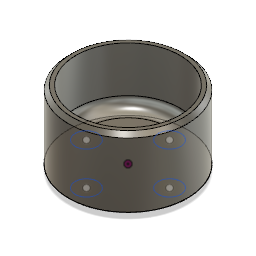
candle_holder (Autodesk Fusion 360 design; units mm, degrees)
Autodesk Fusion 360 part; units mm, degrees
note: some values were not read from the file. Set by a fixed rule: which face or edge a step refers to.
sketch "Sketch1" plane through (0, 0, 0) normal (0, 1, 0) x (1, 0, 0)
  circle A0 centre (0, 0) radius 31.75
  dimension "d6" = 63.5
  measures "d6" diameter of A0
extrude "Extrude1" add sketch "Sketch1" along normal blind 36.45
shell "Shell1" thickness 4 removed faces 1 at (9.3307, 36.45, -9.8517)
extrude "Extrude2" add 1 faces at (10.1601, 4, -12.1449) along direction (0, 1, 0) blind 2
fillet "Fillet1" radius 6 1 edges at (-25.8721, 6, -10.0348)
chamfer "Chamfer1" distance 2 angle 45 1 edges at (-29.6014, 36.45, 11.4813)
ref_plane "WorkPlane1" through (0, 0, 0) normal (0, -1, 0) x (-1, 0, 0)
sketch "Sketch2" plane through (0, 0, 0) normal (0, -1, 0) x (1, 0, 0)
  circle A0 centre (-22.225, 0) radius 6
  circle A1 centre (0, -22.225) radius 6
  circle A2 centre (22.225, 0) radius 6
  circle A3 centre (0, 22.225) radius 6
  dimension "d17" = 12
  dimension "d18" = 22.225
  dimension "d20" = 360
  measures "d17" diameter of A0
extrude "Extrude3" add sketch "Sketch2" along normal blind 3.175
sketch "Sketch3" plane through (0, 0, 0) normal (0, 1, 0) x (1, 0, 0)
equation "radius = 31.75 mm"
equation "height = 34.45 mm + bottom_extra_thickness"
equation "d6 = radius * 2"
equation "d7 = height"
equation "thickness = 4 mm"
equation "bottom_extra_thickness = 2 mm"
equation "d12 = bottom_extra_thickness"
equation "d17 = stand_off_radius * 6"
equation "d18 = radius * 0.7"
equation "stand_off_radius = 2 mm"
equation "stand_off_height = ( 1 / 16 ) * 1 in"
equation "d23 = stand_off_height * 2"
